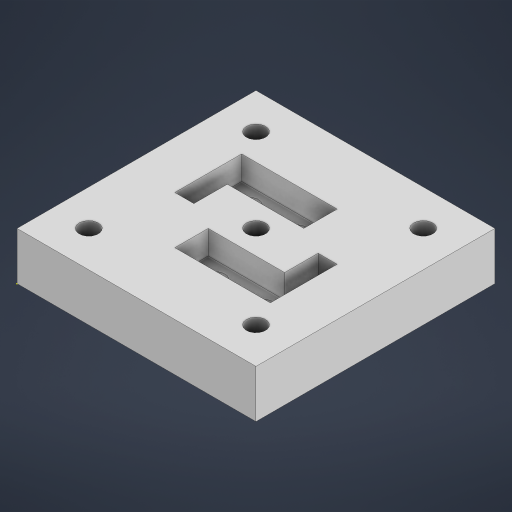
# Autodesk Inventor part: 2_inner_leg_top_plate
Saved by Autodesk Inventor 2024 (Build 280153000, 153)
## iProperties
Created: 2023-05-23
Part Number: 2_inner_leg_top_plate
Material: Generic
Document SubType Name: Modeling
Designer: aasmu
Density: 1 g/cm^3
Appearance: Default
Author: aasmu
Autodesk Inventor part; units mm, degrees
ref_plane "YZ Plane" through (0, 0, 0) normal (1, 0, 0) x (0, 1, 0)
ref_plane "XZ Plane" through (0, 0, 0) normal (0, 1, 0) x (-1, 0, 0)
ref_plane "XY Plane" through (0, 0, 0) normal (0, 0, 1) x (1, 0, 0)
sketch "Sketch1" plane through (0, 0, 0) normal (0, 1, 0) x (-1, 0, 0)
  point P0 (0, 0)
sketch "Sketch2" plane through (0, 0, 0) normal (0, 1, 0) x (-1, 0, 0)
  line L0 (0, 0) -> (-50, 0)
  line L1 (-50, 0) -> (-50, -50)
  line L2 (-50, -50) -> (0, -50)
  line L3 (0, -50) -> (0, 0)
  line L4 (0, -25) -> (-11.3835, -25)
  line L5 (-25, -50) -> (-25, 0)
  circle A0 centre (-7.5, -42.5) radius 2
  circle A1 centre (-7.5, -7.5) radius 2
  line L6 (-7.5, -42.5) -> (-7.5, -50)
  line L7 (-7.5, -7.5) -> (-7.5, 0)
  line L8 (-7.5, -42.5) -> (0, -42.5)
  line L9 (-10, -27) -> (-14, -27)
  line L10 (-14, -27) -> (-14, -23)
  line L11 (-14, -23) -> (-10, -23)
  line L12 (-10, -23) -> (-10, -27)
  circle A2 centre (-42.5, -42.5) radius 2
  circle A3 centre (-42.5, -7.5) radius 2
  line L13 (-40, -27) -> (-36, -27)
  line L14 (-36, -27) -> (-36, -23)
  line L15 (-36, -23) -> (-40, -23)
  line L16 (-40, -23) -> (-40, -27)
  circle A4 centre (-25, -25) radius 2
  line L17 (-14, -27) -> (-14, -30)
  line L18 (-14, -30) -> (-30, -30)
  line L19 (-30, -30) -> (-30, -37)
  line L20 (-30, -37) -> (-10, -37)
  line L21 (-10, -37) -> (-10, -27)
  line L22 (-40, -23) -> (-40, -13)
  line L23 (-40, -13) -> (-20, -13)
  line L24 (-20, -13) -> (-20, -20)
  line L25 (-20, -20) -> (-36, -20)
  line L26 (-36, -20) -> (-36, -23)
  line L27 (-30, -33.5) -> (-10, -33.5)
  line L28 (-20, -16.5) -> (-40, -16.5)
  circle A5 centre (-25, -33.5) radius 2
  circle A6 centre (-15, -33.5) radius 2
  circle A7 centre (-25, -16.5) radius 2
  circle A8 centre (-35, -16.5) radius 2
  point P0 (-10, -25)
  point P1 (-40, -25)
  dimension "d0" = 50
  dimension "d1" = 4
  dimension "d2" = 35
  dimension "d6" = 4
  dimension "d7" = 10
  dimension "d8" = 4
  dimension "d9" = 10
  dimension "d10" = 7
  dimension "d11" = 20
  dimension "d12" = 10
  dimension "d13" = 10
  dimension "d14" = 4
  dimension "d15" = 4
  dimension "d16" = 4
  dimension "d17" = 4
  constraints: 58 end point, 12 perpendicular, 12 point on line, 9 centre point, 7 equal length, 7 midpoint, 7 symmetric about line, 5 coincident, 4 horizontal, 4 parallel, 3 vertical, 2 collinear, 1 equal radius, 2 other
  measures "d0" distance of L2.end L0.start
  measures "d1" diameter of A0
  measures "d2" distance of L7.start L6.start
  measures "d6" distance of L9.end L10.end
  measures "d7" distance of point (-10, -25) L4.start
  measures "d8" diameter of A4
  measures "d9" distance of L20.end L9.start
  measures "d10" distance of L18.end L19.end
  measures "d11" distance of L19.end L20.end
  measures "d12" distance of point (-25, -33.5) point (-15, -33.5)
  measures "d13" distance of point (-35, -16.5) point (-25, -16.5)
  measures "d14" diameter of A5
  measures "d15" diameter of A6
  measures "d16" diameter of A7
  measures "d17" diameter of A8
extrude "Extrusion1" add sketch "Sketch2" along normal blind 10 contours L3 L4 L12 L11 L10 L17 L18 L5 A4 L25 L24 L23 L0 | L3 L8 A0 L6 L2 L5 L20 L21 L12 L4 | L5 L23 L22 L16 L13 L14 L26 L25 A4 L18 L19 L20 L2 L1 L0 | L3 L2 L6 A0 L8
extrude "Extrusion2" add sketch "Sketch2" along normal blind 5 contours L23 L24 L28 A7 L5 | L5 A7 L28 A8 L22 L23 | L21 L27 A6 A5 L5 L18 L17 L9 | L21 L20 L5 A5 L27 A6 | L28 L24 L25 L5 A7 | A7 L5 L25 L26 L15 L22 L28 A8 | L20 L19 L27 A5 L5 | L5 A5 L27 L19 L18
fillet "Fillet1" radius 2 2 edges at (12, 5, -27) (38, 5, -23)
equation "\"d0\" = width"
equation "\"d1\" = screw_hole_diameter"
equation "\"d2\" = hole_spacing"
equation "\"d6\" = cabel_channel_depth"
equation "\"d7\" = rail_depth"
equation "\"d8\" = screw_hole_diameter"
equation "\"d18\" = plate_thicknes"
equation "\"d20\" = 0.5 * plate_thicknes"
equation "\"plate_thicknes\" = 10"
equation "\"width\" = 50"
equation "\"screw_hole_diameter\" = 4"
equation "\"hole_spacing\" = 35"
equation "\"cabel_channel_depth\" = 4"
equation "\"rail_depth\" = 10"
body "Solid1"
